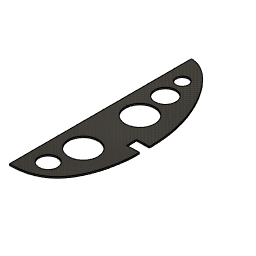
heckfinne_DLG (Autodesk Fusion 360 design; units mm, degrees)
Autodesk Fusion 360 part; units mm, degrees
sketch "Skizze1" plane through (0, 0, 0) normal (0, 1, 0) x (1, 0, 0)
  line L0 (0, 107.5) -> (0, -107.5)
  line L1 (50.4279, -19.4927) -> (65, -18.9838)
  line L2 (50.4279, -19.4927) -> (50.0091, -7.5)
  line L3 (50.0091, -7.5) -> (65, -6.9765)
  line L4 (0, 0) -> (59.8475, 0) construction
  spline S0 degree 5 poles (0, -107.5) (6.9963, -107.5) (19.7475, -106.2356) (35.1536, -100.5492) (49.2456, -86.624) (59.4624, -63.5268) (63.6472, -44.237) (65.0113, -30.9473) (65.1348, -22.8452) (65, -18.9838) knots 0 0 0 0 0 0 0.2 0.4 0.6 0.8 1 1 1 1 1 1
  line L5 (65.2619, -26.4838) -> (64.7381, -11.4838)
  line L6 (-12.5, -107.5) -> (12.5, -107.5)
  spline S1 degree 5 poles (0, 107.5) (3.4735, 107.5) (10.463, 106.2697) (21.0748, 100.7368) (35.1986, 86.9145) (51.0909, 61.8673) (60.389, 37.1064) (64.1612, 16.0697) (65, 0.897) (65, -6.9765) knots 0 0 0 0 0 0 0.2 0.4 0.6 0.8 1 1 1 1 1 1
  line L7 (-7.5, 107.5) -> (7.5, 107.5)
  line L8 (65, 13.0235) -> (65, -26.9765)
  dimension "d1" = 215
  dimension "d2" = 107.5
  dimension "d4" = 65
  dimension "d5" = 15
  dimension "d7" = 12
  dimension "d8" = 15
  dimension "d9" = 25
  dimension "d10" = 40
  dimension "d11" = 15
  dimension "d12" = 100
  dimension "d13" = 2
  constraint vertical L0
  constraint coincident L4.start L0
  constraint perpendicular L1 L2
  constraint perpendicular L2 L3
  constraint coincident L4.start origin
  constraint perpendicular L0 L4
  constraint vertical L1.end L3.end
  constraint midpoint L1.end L5
  constraint perpendicular L1 L5
  constraint midpoint L0.end L6
  constraint perpendicular L0 L6
  constraint midpoint L0.start L7
  constraint perpendicular L0 L7
  constraint midpoint L3.end L8
  constraint coincident L1.end L8
  measures "d1" distance of L0.start L0.end
  measures "d2" distance of L4.start L0.start
  measures "d4" horizontal distance of L4.start L3.end
  measures "d5" distance of L2.end L3.end
  measures "d7" distance of L1 L3
  measures "d8" distance of L7.start L7.end
  measures "d9" distance of L6.start L6.end
  measures "d10" distance of L8.start L8.end
  measures "d11" vertical distance of L5.start L5.end
  measures "d12" vertical distance of L0.end L2.end
  measures "d13" angle of L3 L4
extrude "Extrusion1" add sketch "Skizze1" along normal blind 1.5 contours L0 L1 L2 L3 S0 S1 L8 | S0 L8
sketch "Skizze2" plane through (0, 1.5, 0) normal (0, 1, 0) x (-1, 0, 0)
  spline S0 degree 5 poles (0, 107.5) (-6.9963, 107.5) (-19.7475, 106.2356) (-35.1536, 100.5492) (-49.2456, 86.624) (-59.4624, 63.5268) (-63.6472, 44.237) (-65.0113, 30.9473) (-65.1348, 22.8452) (-65, 18.9838) knots 0 0 0 0 0 0 0.2 0.4 0.6 0.8 1 1 1 1 1 1
  line L0 (-65, 18.9838) -> (-50.4279, 19.4927)
  line L1 (-50.4279, 19.4927) -> (-50.0091, 7.5)
  line L2 (-50.0091, 7.5) -> (-65, 6.9765)
  spline S1 degree 5 poles (-65, 6.9765) (-65, -0.897) (-64.1612, -16.0697) (-60.389, -37.1064) (-51.0909, -61.8673) (-35.1986, -86.9145) (-21.0748, -100.7368) (-10.463, -106.2697) (-3.4735, -107.5) (0, -107.5) knots -1 -1 -1 -1 -1 -1 -0.8 -0.6 -0.4 -0.2 0 0 0 0 0 0
  line L3 (0, -107.5) -> (0, 107.5)
  line L4 (-10, -105.5059) -> (-10, 106.9256) construction
  line L5 (-64.7198, -3.0198) -> (0, -0.7597) construction
  line L6 (-64.8519, 28.9951) -> (0, 31.2598) construction
  circle A0 centre (-27.5, -19.2307) radius 17.5
  circle A1 centre (-22.5, -54.2307) radius 12.5
  circle A2 centre (-17.5, -79.2307) radius 7.5
  circle A3 centre (-27.5, 47.8101) radius 17.5
  circle A4 centre (-21, 82.8101) radius 11
  dimension "d16" = 10
  dimension "d17" = 10
  dimension "d18" = 10
  dimension "d19" = 35
  dimension "d20" = 25
  dimension "d21" = 35
  dimension "d22" = 15
  dimension "d23" = 25
  dimension "d24" = 35
  dimension "d25" = 35
  dimension "d28" = 22
  constraint coincident S1 L4.start
  constraint coincident S0 L4.end
  constraint vertical L4
  constraint coincident S1 L5.start
  constraint coincident L3 L5.end
  constraint parallel L2 L5
  constraint coincident S0 L6.start
  constraint coincident L3 L6.end
  constraint parallel L0 L6
  constraint tangent L4 A0
  constraint tangent L5 A0
  constraint tangent L4 A1
  constraint tangent L4 A2
  constraint tangent L6 A3
  constraint tangent L4 A3
  constraint tangent L4 A4
  measures "d16" distance of L3 L4
  measures "d17" distance of L2 L5
  measures "d18" distance of L0 L6
  measures "d19" diameter of A0
  measures "d20" diameter of A1
  measures "d21" vertical distance of A0.centre A1.centre
  measures "d22" diameter of A2
  measures "d23" vertical distance of A1.centre A2.centre
  measures "d24" diameter of A3
  measures "d25" vertical distance of A3.centre A4.centre
  measures "d28" diameter of A4
extrude "Extrusion2" cut sketch "Skizze2" against normal blind 5 contours A0 | A1 | A2 | A3 | A4
equation "d2 = d1 / 2"
equation "d18 = d17"
